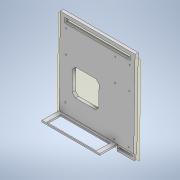
# Autodesk Inventor part: Case-01
Saved by Autodesk Inventor 2020 (Build 240168000, 168)
## iProperties
Created: 2026-07-11
Part Number: Case-01
Material: Generic
Document SubType Name: Modeling
Designer: Nessa
Density: 1 g/cm^3
Appearance: Default
Mass: 599.509 g
Surface Area: 1303.24 cm^2
Volume: 599.509 cm^3
Author: Nessa
## iProperties of the stored document _3DPrint.ipt
Created: 2026-07-11
Part Number: _3DPrint
Material: Generic
Document SubType Name: Modeling
Designer: Nessa
Density: 1 g/cm^3
Appearance: Default
Author: Nessa
Autodesk Inventor part; units mm, degrees
ref_plane "YZ Plane" through (0, 0, 0) normal (1, 0, 0) x (0, 1, 0)
ref_plane "XZ Plane" through (0, 0, 0) normal (0, 1, 0) x (-1, 0, 0)
ref_plane "XY Plane" through (0, 0, 0) normal (0, 0, 1) x (1, 0, 0)
sketch "Sketch1" plane through (0, 0, 0) normal (0, 0, 1) x (1, 0, 0)
  line L0 (-125, 120) -> (125, 120)
  line L1 (125, 120) -> (125, -120)
  line L2 (125, -120) -> (-125, -120)
  line L3 (-125, -120) -> (-125, 120)
  point P0 (0, 0)
  dimension "d0" = 250
  dimension "d1" = 240
  dimension "d2" = 125
  dimension "d3" = 120
  constraints: 8 end point, 2 parallel, 1 horizontal, 1 perpendicular
  measures "d0" distance of L1.end L2.end
  measures "d1" distance of L0.end L1.end
  measures "d2" distance from line of L3 point (0, 0)
  measures "d3" distance from line of L0 point (0, 0)
extrude "Extrusion1" add sketch "Sketch1" along normal mid plane 10
sketch "Sketch5" plane through (0, 0, 5) normal (0, 0, 1) x (1, 0, 0)
  line L0 (-115, 100) -> (-115, -103.2)
  line L1 (-92.14, 100) -> (-92.14, -103.2)
  line L2 (39.94, 100) -> (39.94, -103.2)
  line L3 (112.33, 100) -> (112.33, -103.2)
  line L4 (-92.14, 100) -> (112.33, 100)
  line L5 (-115, -57.48) -> (39.94, -57.48)
  line L6 (112.33, -57.48) -> (39.94, -57.48)
  line L7 (-115, -103.2) -> (39.94, -103.2)
  line L8 (112.33, -103.2) -> (39.94, -103.2)
  line L9 (-115, 100) -> (-92.14, 100)
  line L10 (-125, 120) -> (-125, -120) projected
  line L11 (125, 120) -> (-125, 120) projected
  point P0 (0, 0)
  dimension "d25" = 10
  dimension "d26" = 22.86
  dimension "d27" = 72.39
  dimension "d28" = 132.08
  dimension "d29" = 45.72
  dimension "d30" = 157.48
  dimension "d38" = 20
  constraints: 20 end point, 6 point on line, 4 perpendicular, 4 vertical, 2 collinear, 1 horizontal, 1 parallel
  measures "d25" distance between parallel lines of L10 L0
  measures "d26" distance between parallel lines of L1 L0
  measures "d27" distance between parallel lines of L3 L2
  measures "d28" distance between parallel lines of L2 L1
  measures "d29" distance between parallel lines of L8 L6
  measures "d30" distance between parallel lines of L4 L6
  measures "d38" distance between parallel lines of L11 L4
hole "Hole2" at (-92.14, 100, 5) at (39.94, 100, 5) at (112.33, 100, 5) at (112.33, -57.48, 5) at (39.94, -57.48, 5) at (39.94, -103.2, 5) at (112.33, -103.2, 5) at (-115, -57.48, 5) at (-115, -103.2, 5) direction (0, 0, -1) diameter 3.6 depth 5 tip angle 118
thicken "Thicken1" operation add thickness 5 both sides no extend neighbours yes toward (-1, 0, 0) faces at (-125, 40, -1.6667)
sketch "Sketch11" plane through (0, 0, 5) normal (0, 0, 1) x (1, 0, 0)
  line L0 (125, 120) -> (-130, 120) projected
  line L1 (-130, -120) -> (125, -120) projected
  line L2 (-130, 120) -> (-125, 120)
  line L3 (-125, 120) -> (-125, -120)
  line L4 (-125, -120) -> (-130, -120)
  line L5 (-130, -120) -> (-130, 120)
  point P0 (0, 0)
  dimension "d70" = 5
  constraints: 8 end point, 2 parallel, 1 horizontal, 1 perpendicular, 1 point on line
  measures "d70" distance of L3.end L4.end
extrude "Extrusion5" add sketch "Sketch11" along normal blind 55
sketch "Sketch12" plane through (-130, -120, -5) normal (-1, 0, 0) x (0, 0, 1)
  line L0 (10, 221.8) -> (10, 218.2) projected
  line L1 (10, 220) -> (65, 220)
  line L2 (65, 240) -> (65, 0) projected
  line L3 (62.32, 226.75) -> (17.62, 226.75)
  line L4 (17.62, 226.75) -> (17.62, 67.75)
  line L5 (17.62, 67.75) -> (62.32, 67.75)
  line L6 (62.32, 67.75) -> (62.32, 226.75)
  line L7 (10, 240) -> (10, 0) projected
  line L8 (10, 0) -> (10, 240) projected
  line L9 (65, 0) -> (65, 240) projected
  line L10 (10, 54.5) -> (65, 54.5)
  line L11 (65, 54.5) -> (65, 0)
  line L12 (65, 0) -> (10, 0)
  line L13 (10, 0) -> (10, 54.5)
  point P0 (10, 0)
  point P1 (65, 54.5)
  point P2 (10, 54.5)
  dimension "d75" = 44.7
  dimension "d76" = 159
  dimension "d77" = 6.75
  dimension "d78" = 7.62
  dimension "d79" = 13.25
  constraints: 18 end point, 4 parallel, 3 horizontal, 2 perpendicular, 2 point on line, 1 midpoint
  measures "d75" distance of L5.end L4.end
  measures "d76" distance of L4.end L3.end
  measures "d77" distance between parallel lines of L3 L1
  measures "d78" distance between parallel lines of L7 L4
  measures "d79" distance between parallel lines of L10 L5
extrude "Extrusion6" cut sketch "Sketch12" against normal up to surface (5 mm away) contours L4 L3 L6 L1 | L1 L6 L5 L4 | L10 L2 L12 L7
ref_plane "Work Plane1" through (0, 0, -1.42) normal (0, 0, 1) x (1, 0, 0)
sketch "Sketch13" plane through (0, 0, -1.42) normal (0, 0, 1) x (1, 0, 0)
  line L0 (-130, -120) -> (-130, -65.5) projected
  line L1 (-130, -65.5) -> (-145, -65.5)
  line L2 (-145, -65.5) -> (-145, -120)
  line L3 (-145, -120) -> (-130, -120)
  line L4 (-130, -120) -> (-130, -65.5)
  point P0 (0, 0)
  dimension "d83" = 15
  dimension "d86" = 54.5
  constraints: 8 end point, 2 parallel, 1 horizontal, 1 perpendicular
  measures "d83" distance of L3.end L2.end
  measures "d86" distance between parallel lines of L3 L1
extrude "Extrusion7" add sketch "Sketch13" along normal blind 5
sketch "Sketch14" plane through (0, 0, 3.58) normal (0, 0, 1) x (1, 0, 0)
  line L0 (-145, -120) -> (-130, -120) projected
  line L1 (-131.22, -72.75) -> (-136.22, -72.75)
  line L2 (-136.22, -72.75) -> (-136.22, -112.75)
  line L3 (-136.22, -112.75) -> (-131.22, -112.75)
  line L4 (-131.22, -112.75) -> (-131.22, -72.75)
  line L5 (-130, -120) -> (-130, -65.5) projected
  line L6 (-125, 120) -> (-125, -65.5) projected
  circle A0 centre (-133.72, -72.75) radius 2.5
  circle A1 centre (-133.72, -112.75) radius 2.5
  point P0 (0, 0)
  point P1 (-137.2605, -92.75)
  dimension "d87" = 27.25
  dimension "d88" = 5
  dimension "d89" = 40
  dimension "d90" = 20
  dimension "d92" = 6.22
  constraints: 8 end point, 2 centre point, 2 midpoint, 2 parallel, 2 tangent, 1 horizontal, 1 perpendicular
  measures "d87" distance from line of L0 point (-137.26, -92.75)
  measures "d88" distance of L3.end L2.end
  measures "d89" distance of L2.end L1.end
  measures "d90" distance from line of L3 point (-137.26, -92.75)
  measures "d92" distance between parallel lines of L4 L6
extrude "Extrusion8" cut sketch "Sketch14" against normal up to surface (5 mm away)
sketch "Sketch15" plane through (0, 0, 5) normal (0, 0, 1) x (1, 0, 0)
  line L0 (-125, 120) -> (-125, -65.5) projected
  line L1 (-145, -120) -> (-130, -120) projected
  line L2 (-125, -65.5) -> (-130, -65.5)
  line L3 (-130, -65.5) -> (-130, -120)
  line L4 (-130, -120) -> (-125, -120)
  line L5 (-125, -120) -> (-125, -65.5)
  point P0 (0, 0)
  constraints: 8 end point, 2 parallel, 1 horizontal, 1 perpendicular
extrude "Extrusion9" cut sketch "Sketch15" against normal blind 1.42
thicken "Thicken2" operation add thickness 25 both sides no extend neighbours yes toward (1, 0, 0) faces at (125, -40, -1.6667)
sketch "Sketch18" plane through (0, 0, 5) normal (0, 0, 1) x (1, 0, 0)
  line L0 (150, 120) -> (-125, 120) projected
  line L1 (140, 105) -> (125, 105)
  line L2 (125, 105) -> (125, -105)
  line L3 (125, -105) -> (140, -105)
  line L4 (140, -105) -> (140, 105)
  line L5 (150, -120) -> (150, 120) projected
  line L6 (20.8941, 78.5076) -> (-64.1059, 78.5076)
  line L7 (-64.1059, 78.5076) -> (-64.1059, -6.4924)
  line L8 (-64.1059, -6.4924) -> (20.8941, -6.4924)
  line L9 (20.8941, -6.4924) -> (20.8941, 78.5076)
  point P0 (0, 0)
  point P1 (139.9053, 0)
  dimension "d102" = 120
  dimension "d103" = 15
  dimension "d104" = 210
  dimension "d105" = 105
  dimension "d106" = 10
  dimension "d107" = 85
  dimension "d108" = 85
  constraints: 16 end point, 4 parallel, 2 horizontal, 2 perpendicular
  measures "d102" distance from line of L0 point (139.905, 0)
  measures "d103" distance of L3.end L2.end
  measures "d104" distance of L2.end L1.end
  measures "d105" distance from line of L3 point (139.905, 0)
  measures "d106" distance between parallel lines of L5 L4
  measures "d107" distance of L8.end L7.end
  measures "d108" distance of L7.end L6.end
extrude "Extrusion11" cut sketch "Sketch18" against normal up to surface (10 mm away)
chamfer "Chamfer4" distance 10 angle 45 4 edges at (-64.1059, 78.5076, 0) (-64.1059, -6.4924, 0) (20.8941, -6.4924, 0) (20.8941, 78.5076, 0)
equation "\"d2\" = 0.5 * d0"
equation "\"d3\" = 0.5 * d1"
equation "\"d87\" = 0.5 * d86"
equation "\"d90\" = 0.5 * d89"
body "Solid1"
